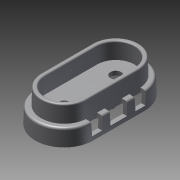
# Autodesk Inventor part: 276-2243
Saved by Autodesk Inventor 2013 (Build 170138000, 138)
## iProperties
Category: Power
Company: Autodesk Inc.
Created: 2012-02-06
Part Number: 276-2243
Document SubType Name: Modeling
Designer: Autodesk Inc.
Density: 1.06 g/cm^3
Catalog Web Link: http://www.vexrobotics.com/276-2243.html
Vendor: VEX
Material: ABS Plastic
Mass: 0.755304 g
Surface Area: 15.3998 cm^2
Volume: 0.712551 cm^3
Author: Autodesk Inc.
Autodesk Inventor part; units mm, degrees
sketch "Sketch1" plane through (0, 0, 0) normal (0, 0, 1) x (1, 0, 0)
  arc A0 (-6.25, 7) -> (-6.25, -7) centre (-6.25, 0) ccw
  line L0 (6.25, -7) -> (-6.25, -7)
  arc A1 (6.25, -7) -> (6.25, 7) centre (6.25, 0) ccw
  line L1 (-6.25, 7) -> (6.25, 7)
  arc A2 (-6.25, 5.999657) -> (-6.25, -5.999657) centre (-6.25, 0) ccw
  line L2 (-6.25, 5.999657) -> (6.25, 5.999657)
  arc A3 (6.25, -5.999657) -> (6.25, 5.999657) centre (6.25, 0) ccw
  line L3 (6.25, -5.999657) -> (-6.25, -5.999657)
  point P0 (0, 0)
  point P1 (0, 0)
  constraints: 8 end point, 8 point on circle, 4 centre point
sketch "Sketch1 outline for Extrusion1" plane through (0, 0, 0) normal (0, 0, 1) x (1, 0, 0)
  line L0 (6.25, 7) -> (-6.25, 7)
  arc A0 (6.25, -7) -> (6.25, 7) centre (6.25, 0) ccw
  line L1 (-6.25, -7) -> (6.25, -7)
  arc A1 (-6.25, 7) -> (-6.25, -7) centre (-6.25, 0) ccw
extrude "Extrusion1" add sketch "Sketch1 outline for Extrusion1" against normal blind 3.9878 draft -1.5
extrude "Extrusion2" cut sketch "Sketch1" against normal blind 2.9972 draft -0.5 contours L2 A3 L3 A2
sketch "Sketch2" plane through (0, 0, -3.9878) normal (0, 0, -1) x (-1, 0, 0)
  arc A0 (-6.607223, 5.593348) -> (-6.607223, -5.593348) centre (-6.25, 0) ccw
  line L0 (6.25, 5.604744) -> (-3.892777, 5.604744)
  arc A1 (6.607223, -5.593348) -> (6.25, 5.604744) centre (6.25, 0) ccw
  line L1 (2.104762, -5.604744) -> (3.892777, -5.604744)
  line L2 (3.892777, -5.604744) -> (6.25, -5.604744)
  arc A2 (6.25, -5.604744) -> (6.607223, -5.593348) centre (6.25, 0) ccw
  line L3 (-2.104762, -5.604744) -> (2.104762, -5.604744)
  line L4 (-3.892777, -5.604744) -> (-2.104762, -5.604744)
  line L5 (-6.25, -5.604744) -> (-3.892777, -5.604744)
  arc A3 (-6.607223, -5.593348) -> (-6.25, -5.604744) centre (-6.25, 0) ccw
  arc A4 (-6.25, 5.604744) -> (-6.607223, 5.593348) centre (-6.25, 0) ccw
  line L6 (-3.892777, 5.604744) -> (-6.25, 5.604744)
  point P0 (0, 0)
  point P1 (-6.607223, 6.398213)
  point P2 (-6.607223, -6.398213)
  point P3 (0, 0)
  constraints: 14 end point, 10 point on circle, 5 centre point
extrude "Extrusion3" add sketch "Sketch2" along normal blind 3.9878 draft -1.5
ref_plane "Work Plane1" through (0, 0, -3.9878) normal (0, 0, -1) x (-1, 0, 0)
sketch "Sketch3" plane through (0, 0, -3.9878) normal (0, 0, -1) x (-1, 0, 0)
  arc A0 (6.25, -4.5) -> (6.25, 4.5) centre (6.25, 0) ccw
  line L0 (6.25, 4.5) -> (-6.25, 4.5)
  arc A1 (-6.25, 4.5) -> (-6.25, -4.5) centre (-6.25, 0) ccw
  line L1 (-6.25, -4.5) -> (6.25, -4.5)
  circle A2 centre (6.25, 0) radius 1.3
  circle A3 centre (-6.25, 0) radius 1.3
  point P0 (0, 0)
  point P1 (0, 0)
  constraints: 4 centre point, 4 end point, 4 point on circle
extrude "Extrusion4" cut sketch "Sketch3" along normal up to next contours L1 A1 L0 A0 | A2 | A3
extrude "Extrusion5" cut sketch "Sketch3" against normal up to next contours A2 | A3
sketch "Sketch4" plane through (0, 0, -2.9972) normal (0, 0, 1) x (1, 0, 0)
  circle A0 centre (-2, 2.8) radius 1
  circle A1 centre (3, -2.8) radius 1
  circle A2 centre (2, 2.8) radius 1
  circle A3 centre (-3, -2.8) radius 1
  point P0 (0, 0)
  point P1 (0, 0)
  constraints: 4 centre point
extrude "Extrusion6" add sketch "Sketch4" along normal blind 2.0066
ref_plane "Work Plane2" through (-6.25, 7, 0) normal (0, 1, 0) x (1, 0, 0)
sketch "Sketch5" plane through (-6.25, 7, 0) normal (0, 1, 0) x (1, 0, 0)
  line L0 (0, 0) -> (12.5, 0)
  line L1 (12.7, 1) -> (12.856584, 3.9878)
  line L2 (10.3, 1) -> (12.5, 1)
  line L3 (12.5, 1) -> (12.7, 1)
  line L4 (10.143416, 3.9878) -> (10.3, 1)
  line L5 (8.25, 1) -> (8.354336, 3.9878)
  line L6 (8.25, 1) -> (4.25, 1)
  line L7 (4.145664, 3.9878) -> (4.25, 1)
  line L8 (2.2, 1) -> (2.356584, 3.9878)
  line L9 (-0.356584, 3.9878) -> (-0.2, 1)
  line L10 (-0.2, 1) -> (2.2, 1)
  line L11 (-0.2, 1) -> (-0.331705, 3.513088)
  line L12 (-0.331705, 3.513088) -> (-0.331705, 3.513088)
  line L13 (-0.331705, 3.513088) -> (-0.2, 1)
  line L14 (0, 0) -> (0, 0)
  line L15 (12.7, 1) -> (12.831705, 3.513088)
  line L16 (10.3, 1) -> (10.168295, 3.513088)
  line L17 (12.5, 3.9878) -> (0, 3.9878)
  line L18 (-0.356584, 3.9878) -> (2.356584, 3.9878)
  line L19 (4.145664, 3.9878) -> (8.354336, 3.9878)
  line L20 (10.143416, 3.9878) -> (12.856584, 3.9878)
  point P0 (6.25, 0)
  point P1 (6.25, 0)
  constraints: 40 end point, 8 point on line, 3 collinear
extrude "Extrusion7" cut sketch "Sketch5" against normal up to surface surface through (3.892777, 5.604744, -3.9878) normal (0, 0.9996573, -0.0261769)
ref_plane "Work Plane3" through (6.25, -7, 0) normal (0, 1, 0) x (-1, 0, 0)
sketch "Sketch6" plane through (6.25, -7, 0) normal (0, 1, 0) x (-1, 0, 0)
  line L0 (2.2, -1) -> (2.356584, -3.9878)
  line L1 (0, -1) -> (2.2, -1)
  line L2 (-0.2, -1) -> (-0.356584, -3.9878)
  line L3 (12.856584, -3.9878) -> (12.7, -1)
  line L4 (10.143416, -3.9878) -> (10.3, -1)
  line L5 (10.3, -1) -> (12.5, -1)
  line L6 (12.5, -3.9878) -> (0, -3.9878)
  line L7 (-0.356584, -3.9878) -> (2.356584, -3.9878)
  line L8 (2.356584, -3.9878) -> (2.2, -1)
  line L9 (2.2, -1) -> (-0.2, -1)
  line L10 (-0.356584, -3.9878) -> (-0.2, -1)
  line L11 (10.143416, -3.9878) -> (12.856584, -3.9878)
  line L12 (12.7, -1) -> (12.856584, -3.9878)
  line L13 (12.7, -1) -> (10.3, -1)
  line L14 (10.3, -1) -> (10.143416, -3.9878)
  point P0 (6.25, 0)
  constraints: 16 end point, 6 parallel, 2 collinear
extrude "Extrusion8" cut sketch "Sketch6" along normal up to surface surface through (3.892777, -5.604744, -3.9878) normal (0, -0.9996573, -0.0261769)
fillet "Fillet1" radius 0.508 5 edges at (-13.1456, 0, -3.9878) (-2.9989, 6.8956, -3.9878) (2.9989, 6.8956, -3.9878) (13.1456, 0, -3.9878) (0, -6.8956, -3.9878)
fillet "Fillet2" radius 0.3048 8 edges at (0, 5.5003, -7.9756) (-11.7475, 0.1754, -7.9756) (0, -5.5003, -7.9756) (11.7503, 0, -7.9756) (0, 4.5, -7.9756) (-10.75, 0, -7.9756) (0, -4.5, -7.9756) (10.75, 0, -7.9756)
body "Solid1"
